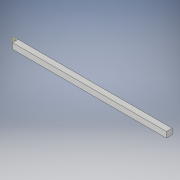
# Autodesk Inventor part: jewlArmBeam
Saved by Autodesk Inventor 2017 (Build 210142000, 142)
## iProperties
Created: 2017-10-14
Part Number: jewlArmBeam
Material: Generic
Document SubType Name: Modeling
Designer: User
Density: 1 g/cm^3
Appearance: Default
Author: User
Autodesk Inventor part; units mm, degrees
ref_plane "YZ Plane" through (0, 0, 0) normal (1, 0, 0) x (0, 1, 0)
ref_plane "XZ Plane" through (0, 0, 0) normal (0, 1, 0) x (-1, 0, 0)
ref_plane "Work Plane1" through (0, 0, 3.175) normal (0, 0, 1) x (1, 0, 0)
sketch "Sketch1" plane through (0, 0, 3.175) normal (0, 0, 1) x (1, 0, 0)
  line L0 (0, 0) -> (342.9, 0)
  line L1 (342.9, 0) -> (342.9, 12.7)
  line L2 (342.9, 12.7) -> (0, 12.7)
  line L3 (0, 12.7) -> (0, 0)
  dimension "d1" = 342.9
  dimension "d2" = 12.7
  constraints: 8 end point, 2 parallel, 1 horizontal, 1 perpendicular
  measures "d1" distance of L2.end L1.end
  measures "d2" distance of L1.end L0.end
extrude "Extrusion1" add sketch "Sketch1" along normal blind 12.7
body "Solid1"
